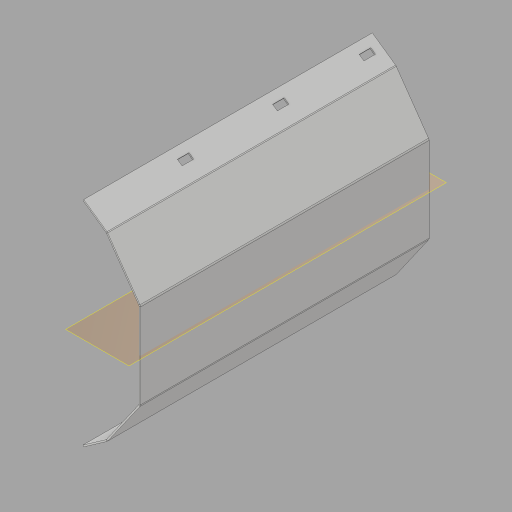
# Autodesk Inventor part: Blech1
Saved by Autodesk Inventor 2023.2 (Build 272271000, 271)
## iProperties
Created: 2023-02-01
Part Number: Blech1
Material: Generisch
Document SubType Name: Sheet Metal
Designer: Raoul Messerli
Density: 1 g/cm^3
Sheet Metal Rule: 5mm
Appearance: Vorgabe
Author: Raoul Messerli
Autodesk Inventor part; units mm, degrees
ref_plane "YZ Plane" through (0, 0, 0) normal (1, 0, 0) x (0, 1, 0)
ref_plane "XZ Plane" through (0, 0, 0) normal (0, 1, 0) x (-1, 0, 0)
sketch "Skizze1" plane through (0, 0, 0) normal (1, 0, 0) x (0, 1, 0)
  line L0 (1000, 150) -> (0, 150)
  line L1 (0, 150) -> (0, -150)
  line L2 (0, -150) -> (1000, -150)
  line L3 (1000, -150) -> (1000, 150)
  point P0 (0, 0)
  point P1 (0, 0)
  dimension "d0" = 1000
  dimension "d1" = 300
  measures "d0" distance of L1.end L2.end
  measures "d1" distance of L2.end L0.start
extrude "Grobblech1" add sketch "Skizze1" along normal blind 5
sketch "Skizze2" plane through (0.9042, 1000, -147.1321) normal (0.819152, 0, -0.5735764) x (0, -1, 0)
  line L0 (1000, 0) -> (0, 0)
  line L1 (0, 0) -> (0, -200)
  line L2 (0, -200) -> (1000, -200)
  line L3 (1000, -200) -> (1000, 0)
  constraints: 6 end point, 1 horizontal, 1 perpendicular, 1 vertical
edge flange "Lasche1" height 200 angle 35 thickness 5 bend radius 5 thickness toward (0.819152, 0, -0.5735764) relief straight relief width 5 relief depth 2.5 edges at (5, 500, -150) wall of the first edge with corners at (0.9042, 0, -147.1321) (0.9042, 1000, -147.1321) (-113.811, 1000, -310.9625) (-113.811, 0, -310.9625)
bend "Biegung1"
corner "Ecke1"
sketch "Skizze3" plane through (-112.5832, 1000, -309.7346) normal (0.5735764, 0, -0.819152) x (0, -1, 0)
  line L0 (1000, 0) -> (0, 0)
  line L1 (0, 0) -> (0, -100)
  line L2 (0, -100) -> (1000, -100)
  line L3 (1000, -100) -> (1000, 0)
  constraints: 6 end point, 1 horizontal, 1 perpendicular, 1 vertical
edge flange "Lasche2" height 100 angle 20 thickness 5 bend radius 5 thickness toward (0.5735764, 0, -0.819152) relief straight relief width 5 relief depth 2.5 edges at (-109.7153, 500, -313.8304) wall of the first edge with corners at (-112.5832, 0, -309.7346) (-112.5832, 1000, -309.7346) (-194.4984, 1000, -367.0923) (-194.4984, 0, -367.0923)
bend "Biegung2"
corner "Ecke2"
sketch "Skizze4" plane through (0.9042, 0, 147.1321) normal (0.819152, 0, 0.5735764) x (0, -1, 0)
  line L0 (-1000, 0) -> (0, 0)
  line L1 (0, 0) -> (0, 200)
  line L2 (0, 200) -> (-1000, 200)
  line L3 (-1000, 200) -> (-1000, 0)
  constraints: 6 end point, 1 horizontal, 1 perpendicular, 1 vertical
edge flange "Lasche3" height 200 angle 35 thickness 5 bend radius 5 thickness toward (0.819152, 0, 0.5735764) relief straight relief width 5 relief depth 2.5 edges at (5, 500, 150) wall of the first edge with corners at (0.9042, 1000, 147.1321) (0.9042, 0, 147.1321) (-113.811, 0, 310.9625) (-113.811, 1000, 310.9625)
bend "Biegung3"
corner "Ecke3"
sketch "Skizze5" plane through (-112.5832, 0, 309.7346) normal (0.5735764, 0, 0.819152) x (0, -1, 0)
  line L0 (-1000, 0) -> (0, 0)
  line L1 (0, 0) -> (0, 100)
  line L2 (0, 100) -> (-1000, 100)
  line L3 (-1000, 100) -> (-1000, 0)
  constraints: 6 end point, 1 horizontal, 1 perpendicular, 1 vertical
edge flange "Lasche4" height 100 angle 20 thickness 5 bend radius 5 thickness toward (0.5735764, 0, 0.819152) relief straight relief width 5 relief depth 2.5 edges at (-109.7153, 500, 313.8304) wall of the first edge with corners at (-112.5832, 1000, 309.7346) (-112.5832, 0, 309.7346) (-194.4984, 0, 367.0923) (-194.4984, 1000, 367.0923)
bend "Biegung4"
corner "Ecke4"
sketch "Skizze7" plane through (-191.6305, 0, 371.1881) normal (0.5735764, 0, 0.819152) x (0.819152, 0, -0.5735764)
  line L0 (98.2367, 1000) -> (0, 1000) projected
  line L1 (30, 1000) -> (30, 0)
  line L2 (0, 0) -> (98.2367, 0) projected
  line L3 (30, 970) -> (50, 970)
  line L4 (50, 970) -> (50, 930)
  line L5 (50, 930) -> (30, 930)
  line L6 (30, 930) -> (30, 970)
  line L7 (30, 670) -> (50, 670)
  line L8 (50, 670) -> (50, 630)
  line L9 (50, 630) -> (30, 630)
  line L10 (30, 630) -> (30, 670)
  line L11 (30, 340) -> (50, 340)
  line L12 (50, 340) -> (50, 300)
  line L13 (50, 300) -> (30, 300)
  line L14 (30, 300) -> (30, 340)
  line L15 (0, 1000) -> (0, 0) projected
  point P0 (369.8792, 0)
  point P1 (40, 670)
  point P2 (30, 950)
  point P3 (30, 930)
  dimension "d45" = 30
  dimension "d46" = 330
  dimension "d47" = 660
  dimension "d48" = 40
  dimension "d49" = 20
  dimension "d50" = 30
  constraints: 26 end point, 7 point on line, 6 parallel, 3 horizontal, 3 perpendicular, 2 collinear, 2 midpoint, 1 vertical
  measures "d45" distance between parallel lines of L3 L0
  measures "d46" distance from line of point (40, 670) L0
  measures "d47" distance between parallel lines of L11 L0
  measures "d48" distance of L3.end L4.end
  measures "d49" distance of L3.start L3.end
  measures "d50" distance from line of point (30, 950) L15
extrude "Extrusion2" cut sketch "Skizze7" against normal through all contours L3 L4 L5 L1 | L7 L8 L9 L1 | L1 L11 L12 L13
mirror "Spiegeln1" about plane through (0, 0, 0) normal (0, 0, 1) of "Extrusion2"
equation "\"d2\" = Stärke"
equation "\"Biegeradius\" = Stärke"
equation "\"MinimalRest\" = 2 * Stärke"
equation "\"Abstandsgröße\" = Stärke"
equation "\"Übergangsradius\" = Biegeradius"
equation "\"JacobiRadiusGröße\" = Biegeradius"
equation "\"GrößeEckenfreistellung\" = 4 * Stärke"
equation "\"TiefeBiegungsfreistellung\" = 0.5 * Stärke"
equation "\"BreiteBiegungsfreistellung\" = Stärke"
equation "\"d3\" = BreiteBiegungsfreistellung"
equation "\"d4\" = TiefeBiegungsfreistellung"
equation "\"d5\" = MinimalRest"
equation "\"d6\" = Übergangsradius"
equation "\"d10\" = GrößeEckenfreistellung"
equation "\"d11\" = Abstandsgröße"
equation "\"d12\" = JacobiRadiusGröße"
equation "\"d13\" = BreiteBiegungsfreistellung"
equation "\"d14\" = TiefeBiegungsfreistellung"
equation "\"d15\" = MinimalRest"
equation "\"d16\" = Übergangsradius"
equation "\"d20\" = GrößeEckenfreistellung"
equation "\"d21\" = Abstandsgröße"
equation "\"d22\" = JacobiRadiusGröße"
equation "\"d23\" = BreiteBiegungsfreistellung"
equation "\"d24\" = TiefeBiegungsfreistellung"
equation "\"d25\" = MinimalRest"
equation "\"d26\" = Übergangsradius"
equation "\"d30\" = GrößeEckenfreistellung"
equation "\"d31\" = Abstandsgröße"
equation "\"d32\" = JacobiRadiusGröße"
equation "\"d33\" = BreiteBiegungsfreistellung"
equation "\"d34\" = TiefeBiegungsfreistellung"
equation "\"d35\" = MinimalRest"
equation "\"d36\" = Übergangsradius"
equation "\"d40\" = GrößeEckenfreistellung"
equation "\"d41\" = Abstandsgröße"
equation "\"d42\" = JacobiRadiusGröße"
equation "\"Stärke\" = 5"
